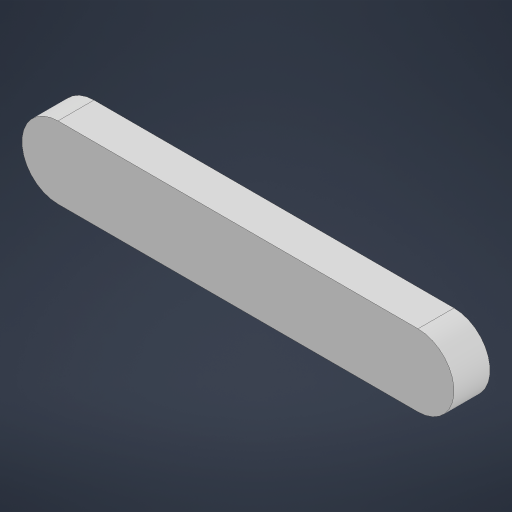
# Autodesk Inventor part: Drone_Latch_Extender
Saved by Autodesk Inventor 2023 (Build 270158000, 158)
## iProperties
Created: 2024-02-27
Part Number: Drone_Latch_Extender
Material: Generic
Document SubType Name: Modeling
Designer: kelle
Density: 1 g/cm^3
Appearance: Default
Author: kelle
Autodesk Inventor part; units mm, degrees
ref_plane "YZ Plane" through (0, 0, 0) normal (1, 0, 0) x (0, 1, 0)
ref_plane "XZ Plane" through (0, 0, 0) normal (0, 1, 0) x (-1, 0, 0)
ref_plane "XY Plane" through (0, 0, 0) normal (0, 0, 1) x (1, 0, 0)
sketch "Sketch1" plane through (0, 0, 0) normal (0, 0, 1) x (1, 0, 0)
  line L0 (15.875, -3.175) -> (-15.875, -3.175)
  line L1 (-15.875, -3.175) -> (-15.875, 3.175)
  line L2 (-15.875, 3.175) -> (15.875, 3.175)
  line L3 (15.875, 3.175) -> (15.875, -3.175)
  line L4 (15.875, -3.175) -> (-15.875, 3.175) construction
  line L5 (-15.875, -3.175) -> (15.875, 3.175) construction
  circle A0 centre (-15.875, 0) radius 3.175
  circle A1 centre (15.875, 0) radius 3.175
  point P0 (0, 0)
  point P1 (15.875, -3.175)
  dimension "d0" = 31.75
  dimension "d1" = 6.35
  constraints: 12 end point, 4 midpoint, 2 parallel, 1 horizontal, 1 perpendicular, 6 other
  measures "d0" distance of L1.end L2.end
  measures "d1" distance of L0.end L1.end
extrude "Extrusion1" add sketch "Sketch1" along normal blind 3.175
body "Solid1"
